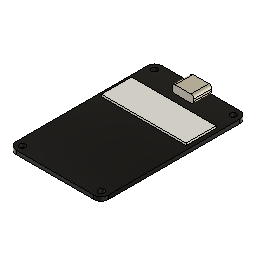
PN532 USB-C v1 (Autodesk Fusion 360 design; units mm, degrees)
Autodesk Fusion 360 part; units mm, degrees
sketch "PCB" plane through (0, 0, 0) normal (0, 0, 1) x (1, 0, 0)
  line L0 (19, -30) -> (-19, -30)
  line L1 (-19, -30) -> (-19, 30)
  line L2 (-19, 30) -> (19, 30)
  line L3 (19, 30) -> (19, -30)
  line L4 (19, -30) -> (-19, 30) construction
  line L5 (-19, -30) -> (19, 30) construction
  dimension "d1" = 38
  dimension "d2" = 60
  constraint horizontal L0
  constraint perpendicular L0 L1
  constraint parallel L0 L2
  constraint parallel L1 L3
  constraint coincident L4 origin
  constraint coincident L5 origin
  measures "d1" distance of L1.end L2.end
  measures "d2" distance of L0.end L1.end
extrude "Extrude1" add sketch "PCB" along normal blind 1.6 makes body 1
sketch "Components & Holes" plane through (0, 0, 1.6) normal (0, 0, 1) x (-1, 0, 0)
  line L0 (-19, -30) -> (19, -30)
  line L1 (19, -30) -> (19, 30)
  line L2 (19, 30) -> (-19, 30)
  line L3 (-19, 30) -> (-19, -30)
  line L4 (4.47, -30) -> (-4.47, -30)
  line L5 (-4.47, -30) -> (-4.47, -22.6)
  line L6 (-4.47, -22.6) -> (4.47, -22.6)
  line L7 (4.47, -22.6) -> (4.47, -30)
  line L8 (0, -30) -> (0, 30) construction
  line L9 (0, -22.6) -> (0, -30) construction
  circle A0 centre (-16.15, -27.15) radius 1.225
  circle A1 centre (-16.15, 27.15) radius 1.225
  circle A2 centre (16.15, 27.15) radius 1.225
  circle A3 centre (16.15, -27.15) radius 1.225
  line L10 (17.375, -18.8) -> (-17.375, -18.8)
  line L11 (-17.375, -18.8) -> (-17.375, -6.5)
  line L12 (-17.375, -6.5) -> (17.375, -6.5)
  line L13 (17.375, -6.5) -> (17.375, -18.8)
  line L14 (17.375, -18.8) -> (-17.375, -6.5) construction
  line L15 (-17.375, -18.8) -> (17.375, -6.5) construction
  point P0 (0, -12.65)
  dimension "d5" = 8.94
  dimension "d6" = 7.4
  dimension "d9" = 2.45
  dimension "d10" = 2.85
  dimension "d11" = 2.85
  dimension "d12" = 2.45
  dimension "d13" = 2.85
  dimension "d14" = 2.85
  dimension "d15" = 34.75
  dimension "d16" = 12.3
  dimension "d17" = 11.2
  constraint horizontal L4
  constraint vertical L5
  constraint horizontal L6
  constraint vertical L7
  constraint collinear L0 L4
  constraint midpoint L0 L8.start
  constraint midpoint L2 L8.end
  constraint midpoint L6 L9.start
  constraint midpoint L4 L8.start
  constraint collinear L8 L9
  constraint symmetric L8 A0 A3
  constraint symmetric L8 A1 A2
  constraint horizontal L10
  constraint perpendicular L10 L11
  constraint parallel L10 L12
  constraint parallel L11 L13
  constraint coincident L14 P0
  constraint coincident L15 P0
  constraint coincident L8 P0
  measures "d5" distance of L4.start L4.end
  measures "d6" distance of L4.start L6.end
  measures "d9" diameter of A0
  measures "d10" distance of L3 A0.centre
  measures "d11" distance of L0 A0.centre
  measures "d12" diameter of A1
  measures "d13" distance of L2 A1.centre
  measures "d14" distance of L3 A1.centre
  measures "d15" distance of L11.end L12.end
  measures "d16" distance of L10.end L11.end
  measures "d17" distance of L0 L10
extrude "Extrude2" add sketch "Components & Holes" along normal blind 3.26 separate body contours L0 L4 L5 L6 L7 makes body 2
extrude "Extrude3" add sketch "Components & Holes" along normal blind 0.9 separate body contours L10 L11 L12 L13 makes body 3
extrude "Extrude4" cut sketch "Components & Holes" against normal up to surface (1.6 mm away) contours A0 | A1 | A2 | A3 bodies 1
fillet "Fillet1" radius 3 4 edges at (19, 30, 0.8) (19, -30, 0.8) (-19, -30, 0.8) (-19, 30, 0.8) on bodies 1
fillet "Fillet2" radius 1.2 4 edges at (4.47, 26.3, 4.86) (-4.47, 26.3, 4.86) (-4.47, 26.3, 1.6) (4.47, 26.3, 1.6) on bodies 2
named bodies: "PCB", "USB-C Socket", "Raised Components"
